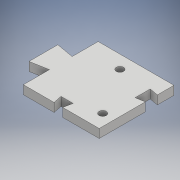
# Autodesk Inventor part: Frame VG01-04
Saved by Autodesk Inventor 2017 (Build 210142000, 142)
## iProperties
Created: 2019-03-04
Part Number: Frame VG01-04
Material: Generic
Document SubType Name: Modeling
Designer: Ben
Density: 1 g/cm^3
Appearance: Default
Author: Ben
Autodesk Inventor part; units mm, degrees
ref_plane "YZ Plane" through (0, 0, 0) normal (1, 0, 0) x (0, 1, 0)
ref_plane "XZ Plane" through (0, 0, 0) normal (0, 1, 0) x (-1, 0, 0)
ref_plane "XY Plane" through (0, 0, 0) normal (0, 0, 1) x (1, 0, 0)
sketch "Sketch1" plane through (0, 0, 0) normal (0, 1, 0) x (-1, 0, 0)
  line L0 (0, 0) -> (0, -35)
  line L1 (0, -35) -> (37, -35)
  line L2 (37, -35) -> (37, -55)
  line L3 (37, -55) -> (48, -55)
  line L4 (48, -55) -> (48, 0)
  line L5 (48, 0) -> (22, 0)
  line L6 (22, 0) -> (22, 0)
  line L7 (22, 0) -> (0, 0)
  dimension "d0" = 35
  dimension "d1" = 37
  dimension "d2" = 20
  dimension "d3" = 11
  dimension "d4" = 55
  dimension "d5" = 26
  dimension "d6" = 0
  constraints: 16 end point, 5 perpendicular, 2 vertical
  measures "d0" distance of L0.start L0.end
  measures "d1" distance of L0.end L1.end
  measures "d2" distance of L1.end L2.end
  measures "d3" distance of L2.end L3.end
  measures "d4" distance of L3.end L4.end
  measures "d5" distance of L4.end L5.end
  measures "d6" distance of L5.end L6.end
extrude "Extrusion1" add sketch "Sketch1" along normal blind 50
shell "Shell1" thickness 5 removed faces 3 at (-48, 16.6667, -36.6667) at (-19.6667, 0, -23.3333) at (-19.6667, 50, -23.3333)
sketch "Sketch2" plane through (0, 0, 0) normal (1, 0, 0) x (0, 0, -1)
  line L0 (5, 0) -> (30, 0) projected
  line L1 (5, 0) -> (19, 0)
  line L2 (19, 0) -> (19, 17)
  line L3 (19, 17) -> (5, 17)
  line L4 (5, 17) -> (5, 0)
  point P0 (0, 0)
  dimension "d10" = 17
  dimension "d11" = 0
  dimension "d12" = 11
  constraints: 8 end point, 2 parallel, 1 horizontal, 1 perpendicular, 1 point on line
  measures "d10" distance of L2.end L1.end
  measures "d11" distance from line of L4 L0.start
  measures "d12" distance from line of L2 L0.end
extrude "Extrusion2" cut sketch "Sketch2" against normal blind 10
sketch "Sketch3" plane through (-48, 0, -55) normal (-1, 0, 0) x (0, 0, 1)
  line L0 (0, 0) -> (0, 50) projected
  line L1 (5, 50) -> (25, 50) projected
  line L2 (0, 0) -> (5, 0)
  line L3 (5, 0) -> (5, 50)
  line L4 (5, 50) -> (0, 50)
  line L5 (0, 50) -> (0, 0)
  point P0 (55, 0)
  constraints: 8 end point, 2 parallel, 1 horizontal, 1 perpendicular
extrude "Extrusion3" add sketch "Sketch3" along normal blind 15
sketch "Sketch4" plane through (-48, 0, 0) normal (-1, 0, 0) x (0, 0, 1)
  line L0 (-5, 0) -> (0, 0) projected
  line L1 (-5, 0) -> (-5, 50) projected
  line L2 (0, 0) -> (-5, 0)
  line L3 (-5, 0) -> (-5, 50)
  line L4 (-5, 50) -> (0, 50)
  line L5 (0, 50) -> (0, 0)
  point P0 (0, 0)
  constraints: 8 end point, 2 parallel, 1 horizontal, 1 perpendicular
extrude "Extrusion4" add sketch "Sketch4" along normal blind 15
sketch "Sketch5" plane through (0, 17, -5) normal (0, 0, -1) x (-1, 0, 0)
  circle A0 centre (11.5, -8.5) radius 2.0828
  line L0 (63, -17) -> (0, -17) projected
  line L1 (0, -17) -> (0, 0) projected
  dimension "d19" = 4.1656
  dimension "d20" = 8.5
  dimension "d21" = 11.5
  constraints: 1 centre point
  measures "d19" diameter of A0
  measures "d20" distance from line of L0 A0.centre
  measures "d21" distance from line of L1 A0.centre
extrude "Extrusion5" cut sketch "Sketch5" against normal blind 15
sketch "Sketch6" plane through (0, 17, -5) normal (0, 0, -1) x (-1, 0, 0)
  circle A0 centre (28.505, 18.46) radius 2.0828
  line L0 (63, -17) -> (0, -17) projected
  line L1 (5, 0) -> (5, 33) projected
  dimension "d24" = 4.1656
  dimension "d25" = 35.46
  dimension "d26" = 23.505
  constraints: 1 centre point
  measures "d24" diameter of A0
  measures "d25" distance from line of L0 A0.centre
  measures "d26" distance from line of L1 A0.centre
extrude "Extrusion6" cut sketch "Sketch6" against normal blind 15
sketch "Sketch7" plane through (0, 17, -5) normal (0, 0, -1) x (-1, 0, 0)
  circle A0 centre (58.5, 19) radius 2.0828
  line L0 (63, 33) -> (63, -17) projected
  line L1 (5, 33) -> (63, 33) projected
  point P0 (0, -17)
  dimension "d29" = 4.1656
  dimension "d30" = 4.5
  dimension "d31" = 14
  constraints: 1 centre point
  measures "d29" diameter of A0
  measures "d30" distance from line of A0.centre L0
  measures "d31" distance from line of L1 A0.centre
extrude "Extrusion7" cut sketch "Sketch7" against normal blind 15
sketch "Sketch13" plane through (0, 0, -35) normal (0, 0, -1) x (-1, 0, 0)
  circle A0 centre (11.5, 8.5) radius 2.0828
  line L0 (0, 0) -> (37, 0) projected
  line L1 (0, 0) -> (0, 50) projected
  dimension "d41" = 4.1656
  dimension "d42" = 8.5
  dimension "d43" = 11.5
  constraints: 1 centre point
  measures "d41" diameter of A0
  measures "d42" distance from line of L0 A0.centre
  measures "d43" distance from line of L1 A0.centre
extrude "Extrusion9" cut sketch "Sketch13" against normal blind 15
sketch "Sketch14" plane through (-37, 0, -55) normal (0, 0, -1) x (-1, 0, 0)
  circle A0 centre (-8.495, 35.46) radius 2.0828
  line L0 (-37, 0) -> (-37, 50) projected
  line L1 (0, 0) -> (26, 0) projected
  dimension "d46" = 4.1656
  dimension "d47" = 28.505
  dimension "d48" = 35.46
  constraints: 1 centre point
  measures "d46" diameter of A0
  measures "d47" distance from line of L0 A0.centre
  measures "d48" distance from line of L1 A0.centre
extrude "Extrusion10" cut sketch "Sketch14" against normal blind 15
sketch "Sketch15" plane through (-37, 0, -55) normal (0, 0, -1) x (-1, 0, 0)
  circle A0 centre (21.5, 36) radius 2.0828
  line L0 (0, 0) -> (26, 0) projected
  line L1 (26, 50) -> (26, 0) projected
  point P0 (-37, 0)
  dimension "d51" = 4.1656
  dimension "d52" = 36
  dimension "d53" = 4.5
  constraints: 1 centre point
  measures "d51" diameter of A0
  measures "d52" distance from line of L0 A0.centre
  measures "d53" distance from line of L1 A0.centre
extrude "Extrusion11" cut sketch "Sketch15" against normal blind 15
sketch "Sketch16" plane through (-42, 0, -30) normal (-1, 0, 0) x (0, 0, 1)
  line L0 (0, 0) -> (-5, 0)
  line L1 (-5, 0) -> (-5, 50)
  line L2 (-5, 50) -> (0, 50)
  line L3 (0, 50) -> (0, 0)
  point P0 (30, 0)
  dimension "d56" = 5
  dimension "d57" = 50
  constraints: 8 end point, 2 parallel, 1 horizontal, 1 perpendicular
  measures "d56" distance of L1.end L2.end
  measures "d57" distance of L0.end L1.end
extrude "Extrusion12" add sketch "Sketch16" along normal blind 21
sketch "Sketch17" plane through (-5, 0, -30) normal (0, 0, 1) x (1, 0, 0)
  circle A0 centre (-23.505, 35.46) radius 2.0828
  line L0 (0, 0) -> (0, 50) projected
  line L1 (0, 0) -> (-58, 0) projected
  point P0 (5, 0)
  dimension "d60" = 4.1656
  dimension "d61" = 23.505
  dimension "d62" = 35.46
  constraints: 1 centre point
  measures "d60" diameter of A0
  measures "d61" distance from line of A0.centre L0
  measures "d62" distance from line of L1 A0.centre
extrude "Extrusion13" cut sketch "Sketch17" against normal blind 10
sketch "Sketch18" plane through (-42, 0, -35) normal (0, 0, -1) x (-1, 0, 0)
  circle A0 centre (16.5, 36) radius 2.0828
  line L0 (21, 50) -> (21, 0) projected
  line L1 (0, 0) -> (21, 0) projected
  point P0 (-42, 0)
  dimension "d65" = 4.1656
  dimension "d67" = 36
  dimension "d70" = 4.5
  constraints: 1 centre point
  measures "d65" diameter of A0
  measures "d67" distance from line of L1 A0.centre
  measures "d70" distance from line of L0 A0.centre
extrude "Extrusion14" cut sketch "Sketch18" against normal blind 10
sketch "Sketch20" plane through (-63, 0, 0) normal (-1, 0, 0) x (0, 0, 1)
  line L0 (0, 0) -> (-5, 0) projected
  line L1 (-5, 17) -> (-5, 50) projected
  line L2 (0, 0) -> (-5, 0)
  line L3 (-5, 0) -> (-5, 50)
  line L4 (-5, 50) -> (0, 50)
  line L5 (0, 50) -> (0, 0)
  constraints: 8 end point, 2 parallel, 1 horizontal, 1 perpendicular
extrude "Extrusion15" add sketch "Sketch20" along normal blind 2.583
sketch "Sketch21" plane through (-63, 0, -30) normal (-1, 0, 0) x (0, 0, 1)
  line L0 (-20, 50) -> (-5, 50) projected
  line L1 (11, 0) -> (0, 0) projected
  line L2 (-5, 50) -> (0, 50)
  line L3 (0, 50) -> (0, 0)
  line L4 (0, 0) -> (-5, 0)
  line L5 (-5, 0) -> (-5, 50)
  point P0 (30, 0)
  constraints: 8 end point, 2 parallel, 1 horizontal, 1 perpendicular
extrude "Extrusion16" add sketch "Sketch21" along normal blind 2.583
sketch "Sketch22" plane through (-63, 0, -55) normal (-1, 0, 0) x (0, 0, 1)
  line L0 (0, 0) -> (0, 50) projected
  line L1 (5, 0) -> (5, 50) projected
  line L2 (0, 50) -> (5, 50)
  line L3 (5, 50) -> (5, 0)
  line L4 (5, 0) -> (0, 0)
  line L5 (0, 0) -> (0, 50)
  point P0 (55, 0)
  constraints: 8 end point, 2 parallel, 1 horizontal, 1 perpendicular
extrude "Extrusion17" add sketch "Sketch22" along normal blind 2.583
sketch "Sketch23" plane through (0, 0, 0) normal (0, 0, 1) x (1, 0, 0)
  line L0 (0, 50) -> (-37, 50) projected
  line L1 (-65.583, 50) -> (-65.583, 0) projected
  line L2 (0, 50) -> (-65.583, 50)
  line L3 (-65.583, 50) -> (-65.583, 43.083)
  line L4 (-65.583, 43.083) -> (0, 43.083)
  line L5 (0, 43.083) -> (0, 50)
  point P0 (0, 0)
  dimension "d77" = 6.917
  constraints: 8 end point, 2 parallel, 1 horizontal, 1 perpendicular, 1 point on line
  measures "d77" distance of L4.end L0.start
extrude "Extrusion18" cut sketch "Sketch23" against normal blind 100
sketch "Sketch24" plane through (0, 0, -35) normal (0, 0, -1) x (-1, 0, 0)
  line L0 (0, 0) -> (65.583, 0) projected
  line L1 (31.0052, 0) -> (26.0052, 0)
  line L2 (26.0052, 5) -> (31.0052, 5)
  circle A0 centre (28.505, 35.46) radius 2.0828 projected
  line L3 (26.0052, 5) -> (25.0052, 5)
  line L4 (25.0052, 5) -> (26.0052, 0)
  line L5 (31.0052, 5) -> (32.0052, 5)
  line L6 (32.0052, 5) -> (31.0052, 0)
  dimension "d80" = 5
  dimension "d81" = 5
  dimension "d83" = 1
  dimension "d84" = 1
  constraints: 12 end point, 3 horizontal, 1 parallel, 1 point on line
  measures "d80" distance of L2.start L2.end
  measures "d81" distance of L1.end L2.start
  measures "d83" distance of L2.start L3.end
  measures "d84" distance of L2.end L5.end
extrude "Extrusion19" cut sketch "Sketch24" against normal blind 100 contours L4 L3 L2 L5 L6 L0
sketch "Sketch25" plane through (-65.583, 0, -55) normal (-1, 0, 0) x (0, 0, 1)
  line L0 (20, 0) -> (0, 0) projected
  line L1 (0, 43.083) -> (20, 43.083) projected
  line L2 (0, 0) -> (5, 0)
  line L3 (5, 0) -> (5, 43.083)
  line L4 (5, 43.083) -> (0, 43.083)
  line L5 (0, 43.083) -> (0, 0)
  point P0 (55, 0)
  dimension "d87" = 5
  constraints: 8 end point, 2 parallel, 1 horizontal, 1 perpendicular, 1 point on line
  measures "d87" distance of L4.end L3.end
extrude "Extrusion20" add sketch "Sketch25" along normal blind 22.5
sketch "Sketch28" plane through (-65.583, 0, -30) normal (-1, 0, 0) x (0, 0, 1)
  line L0 (0, 0) -> (-5, 0) projected
  line L1 (-5, 0) -> (-5, 43.083) projected
  line L2 (0, 0) -> (-5, 0)
  line L3 (-5, 0) -> (-5, 43.083)
  line L4 (-5, 43.083) -> (0, 43.083)
  line L5 (0, 43.083) -> (0, 0)
  point P0 (30, 0)
  constraints: 8 end point, 2 parallel, 1 horizontal, 1 perpendicular
extrude "Extrusion23" add sketch "Sketch28" along normal blind 22.5
sketch "Sketch26" plane through (-37, 0, -55) normal (0, 0, -1) x (-1, 0, 0)
  circle A0 centre (45.232, 36.922) radius 2.0828
  line L0 (51.083, 43.083) -> (51.083, 0) projected
  line L1 (51.083, 43.083) -> (0, 43.083) projected
  point P0 (-37, 0)
  dimension "d90" = 4.1656
  dimension "d91" = 5.851
  dimension "d92" = 6.161
  constraints: 1 centre point
  measures "d90" diameter of A0
  measures "d91" distance from line of L0 A0.centre
  measures "d92" distance from line of L1 A0.centre
extrude "Extrusion21" cut sketch "Sketch26" against normal blind 25
sketch "Sketch27" plane through (-37, 0, -55) normal (0, 0, -1) x (-1, 0, 0)
  circle A0 centre (48.381, 15.906) radius 2.0828
  line L0 (51.083, 43.083) -> (51.083, 0) projected
  line L1 (0, 0) -> (51.083, 0) projected
  point P0 (-37, 0)
  dimension "d95" = 4.1656
  dimension "d96" = 2.702
  dimension "d97" = 15.906
  constraints: 1 centre point
  measures "d95" diameter of A0
  measures "d96" distance from line of L0 A0.centre
  measures "d97" distance from line of A0.centre L1
extrude "Extrusion22" cut sketch "Sketch27" against normal blind 25
sketch "Sketch29" plane through (-42, 0, -35) normal (0, 0, -1) x (-1, 0, 0)
  circle A0 centre (43.381, 15.906) radius 2.0828 projected
  arc A1 (46.083, 19.6075) -> (46.083, 12.2045) centre (43.381, 15.906) ccw
  line L0 (46.083, 43.083) -> (46.083, 0) projected
  line L1 (46.083, 19.6075) -> (46.083, 12.2045)
  point P0 (-42, 0)
  dimension "d102" = 2.5
  constraints: 2 end point, 2 point on circle, 2 point on line, 1 centre point, 1 coincident
  measures "d102" radial gap between concentric circles of A1 A0
extrude "Extrusion24" add sketch "Sketch29" along normal up to next
sketch "Sketch30" plane through (-88.083, 0, -55) normal (-1, 0, 0) x (0, 0, 1)
  line L0 (9, 19.6075) -> (21, 19.6075)
  line L1 (21, 19.6075) -> (21, 5)
  line L2 (21, 5) -> (9, 5)
  line L3 (9, 5) -> (9, 19.6075)
  line L4 (0, 43.083) -> (0, 0) projected
  line L5 (25, 0) -> (25, 43.083) projected
  line L6 (0, 0) -> (5, 0) projected
  line L7 (20, 19.6075) -> (5, 19.6075) projected
  point P0 (55, 0)
  dimension "d105" = 9
  dimension "d106" = 4
  dimension "d107" = 5
  dimension "d108" = 0
  constraints: 8 end point, 2 parallel, 1 horizontal, 1 perpendicular
  measures "d105" distance between parallel lines of L4 L3
  measures "d106" distance between parallel lines of L5 L1
  measures "d107" distance between parallel lines of L6 L2
  measures "d108" distance between parallel lines of L7 L0
extrude "Extrusion25" add sketch "Sketch30" along normal blind 30
sketch "Sketch31" plane through (-88.083, 5, -34) normal (0, 0, 1) x (1, 0, 0)
  circle A0 centre (-23.917, 4) radius 2.0828
  line L0 (-30, 0) -> (-30, 14.6075) projected
  line L1 (0, 0) -> (-30, 0) projected
  point P0 (88.083, -5)
  dimension "d111" = 4.1656
  dimension "d112" = 6.083
  dimension "d113" = 4
  constraints: 1 centre point
  measures "d111" diameter of A0
  measures "d112" distance from line of A0.centre L0
  measures "d113" distance from line of L1 A0.centre
extrude "Extrusion26" cut sketch "Sketch31" against normal blind 30
sketch "Sketch33" plane through (-88.083, 5, -34) normal (0, 0, 1) x (1, 0, 0)
  circle A0 centre (-23.917, 4) radius 2.0828 projected
  arc A1 (-25.0228, 9.9816) -> (-30, 4) centre (-23.917, 4) ccw
  line L0 (-30, 14.6075) -> (-30, 0) projected
  line L1 (-30, 0) -> (-30, 14.6075) projected
  line L2 (0, 14.6075) -> (-30, 14.6075) projected
  line L3 (-30, 4) -> (-30, 14.6075)
  line L4 (0, 14.6075) -> (-30, 14.6075) projected
  line L5 (-30, 14.6075) -> (0, 14.6075)
  line L6 (0, 14.6075) -> (-25.0228, 9.9816)
  point P0 (88.083, -5)
  constraints: 6 end point, 2 point on circle, 2 tangent, 1 centre point, 1 coincident, 1 perpendicular, 1 point on line, 1 vertical
extrude "Extrusion27" cut sketch "Sketch33" against normal blind 30 contours A1 L0 L2 L6
sketch "Sketch34" plane through (-118.083, 5, -34) normal (0, 0, 1) x (1, 0, 0)
  circle A0 centre (6.083, 4) radius 2.0828 projected
  line L0 (0, 0) -> (0, 4) projected
  arc A1 (0, 4) -> (1.5001, 0) centre (6.083, 4) ccw
  line L1 (30, 0) -> (0, 0) projected
  line L2 (1.5001, 0) -> (0, 0)
  arc A2 (4.9772, 9.9816) -> (0, 4) centre (6.083, 4) ccw projected
  line L3 (0, 0) -> (0, 4)
  point P0 (118.083, -5)
  constraints: 4 end point, 2 point on circle, 1 centre point, 1 coincident, 1 collinear, 1 perpendicular, 1 tangent
extrude "Extrusion28" cut sketch "Sketch34" against normal blind 30 contours L0 A1 L1
sketch "Sketch35" plane through (-88.083, 5, -46) normal (0, -1, 0) x (1, 0, 0)
  line L0 (0, 12) -> (0, 11) projected
  line L1 (0, 0) -> (-28.4999, 0) projected
  line L2 (0, 11) -> (0, 0)
  line L3 (0, 0) -> (7.2848, 11)
  line L4 (7.2848, 11) -> (7.2848, -4) projected
  line L5 (0, 11) -> (7.2848, 11)
  line L6 (46.083, 11) -> (0, 11) projected
  point P0 (88.083, 46)
  constraints: 6 end point, 1 collinear, 1 perpendicular, 1 point on line
extrude "Extrusion29" add sketch "Sketch35" against normal up to next
sketch "Sketch36" plane through (0, 0, 0) normal (1, 0, 0) x (0, 0, -1)
  line L0 (30, 43.083) -> (35, 43.083) projected
  line L1 (0, 0) -> (5, 0) projected
  line L2 (30, 43.083) -> (0, 43.083)
  line L3 (0, 43.083) -> (0, 0)
  line L4 (0, 0) -> (30, 0)
  line L5 (30, 0) -> (30, 43.083)
  constraints: 8 end point, 2 parallel, 1 horizontal, 1 perpendicular
extrude "Extrusion30" cut sketch "Sketch36" against normal through all
sketch "Sketch37" plane through (0, 43.083, -35) normal (0, 0, -1) x (-1, 0, 0)
  line L0 (10, -8.694) -> (10, -17.3883)
  line L1 (10, -17.3883) -> (5, -16.5067)
  line L2 (10, -8.694) -> (5, -9.5756)
  line L3 (10, -8.694) -> (15.0771, -8.694) construction
  line L4 (5, -9.5756) -> (5, -16.5067)
  line L5 (0, -43.083) -> (0, 0) projected
  line L6 (0, -43.083) -> (26.0052, -43.083) projected
  dimension "d124" = 8.6943
  dimension "d125" = 80
  dimension "d126" = 170
  dimension "d127" = 5
  dimension "d130" = 5
  dimension "d131" = 34.389
  constraints: 10 end point, 1 equal length, 1 horizontal, 1 parallel
  measures "d124" distance of L0.start L0.end
  measures "d125" angle of L0 L1
  measures "d126" angle of L2 L3
  measures "d127" distance between parallel lines of L0 L4
  measures "d130" distance between parallel lines of L5 L4
  measures "d131" distance from line of L6 L0.start
extrude "Extrusion31" cut sketch "Sketch37" against normal blind 10
sketch "Sketch38" plane through (-37, 0, -35) normal (1, 0, 0) x (0, 0, -1)
  line L0 (20, 43.083) -> (20, 0) projected
  line L1 (0, 0) -> (20, 0)
  line L2 (20, 0) -> (20, 43.083)
  line L3 (20, 43.083) -> (0, 43.083)
  line L4 (0, 43.083) -> (0, 0)
  point P0 (-35, 0)
  constraints: 8 end point, 2 parallel, 1 horizontal, 1 perpendicular
extrude "Extrusion32" cut sketch "Sketch38" against normal through all
sketch "Sketch39" plane through (0, 0, -30) normal (1, 0, 0) x (0, 0, -1)
  line L0 (10, 34.389) -> (10, 25.6947)
  line L1 (10, 25.6947) -> (5, 26.5763)
  line L2 (10, 34.389) -> (5, 33.5074)
  line L3 (10, 34.389) -> (15.0771, 34.389) construction
  line L4 (5, 33.5074) -> (5, 26.5763)
  line L5 (5, 0) -> (5, 43.083) projected
  point P0 (5, 33.5074)
  dimension "d136" = 8.6943
  dimension "d137" = 80
  dimension "d138" = 170
  dimension "d139" = 5
  dimension "d140" = 0
  dimension "d141" = 8.694
  constraints: 10 end point, 1 equal length, 1 horizontal, 1 parallel
  measures "d136" distance of L0.start L0.end
  measures "d137" angle of L0 L1
  measures "d138" angle of L2 L3
  measures "d139" distance between parallel lines of L0 L4
  measures "d140" distance between parallel lines of L5 L4
  measures "d141" vertical distance of L5.end L0.start
extrude "Extrusion33" add sketch "Sketch39" against normal blind 42
sketch "Sketch40" plane through (0, 0, -30) normal (1, 0, 0) x (0, 0, -1)
  line L0 (5, 38.0828) -> (5, 33.9172) projected
  line L1 (5, 36.5278) -> (10.9453, 36.5278)
  line L2 (10.9453, 36.5278) -> (10.9453, 22.5092)
  line L3 (10.9453, 22.5092) -> (5, 22.5092)
  line L4 (5, 22.5092) -> (5, 36.5278)
  point P0 (-30, 0)
  constraints: 8 end point, 2 parallel, 1 horizontal, 1 perpendicular, 1 point on line
extrude "Extrusion34" cut sketch "Sketch40" against normal blind 37
sketch "Sketch41" plane through (0, 0, -35) normal (0, 0, -1) x (-1, 0, 0)
  line L0 (0, 0) -> (5, 0)
  line L1 (5, 0) -> (5, 45.0451)
  line L2 (5, 45.0451) -> (0, 45.0451)
  line L3 (0, 45.0451) -> (0, 0)
  dimension "d146" = 5
  constraints: 8 end point, 2 parallel, 1 horizontal, 1 perpendicular
  measures "d146" distance of L2.end L1.end
extrude "Extrusion35" cut sketch "Sketch41" against normal blind 27
sketch "Sketch43" plane through (-37, 0, -30) normal (1, 0, 0) x (0, 0, -1)
  line L0 (10, 16.9997) -> (10, 8.3054)
  line L1 (10, 8.3054) -> (5, 9.187)
  line L2 (10, 16.9997) -> (5, 16.118)
  line L3 (10, 16.9997) -> (15.0771, 16.9997) construction
  line L4 (5, 16.118) -> (5, 9.187)
  line L5 (10, 34.389) -> (10, 25.6947) projected
  point P0 (5, 0)
  dimension "d149" = 8.6943
  dimension "d150" = 80
  dimension "d151" = 170
  dimension "d152" = 5
  dimension "d153" = 0
  dimension "d154" = 9.187
  constraints: 10 end point, 1 equal length, 1 horizontal, 1 parallel
  measures "d149" distance of L0.start L0.end
  measures "d150" angle of L0 L1
  measures "d151" angle of L2 L3
  measures "d152" distance between parallel lines of L0 L4
  measures "d153" distance between parallel lines of L5 L0
  measures "d154" distance of point (5, 0) L1.end
extrude "Extrusion36" add sketch "Sketch43" against normal blind 5
sketch "Sketch44" plane through (-25.0052, 5, -35) normal (0, 0, -1) x (-1, 0, 0)
  line L0 (23.6844, 38.083) -> (23.6844, 23.083)
  line L1 (23.6844, 23.083) -> (33.6844, 24.8463)
  line L2 (33.6844, 24.8463) -> (33.6844, 8.2367)
  line L3 (33.6844, 8.2367) -> (23.6844, 10)
  line L4 (23.6844, 10) -> (23.6844, -5)
  line L5 (6, -5) -> (63.0778, -5) projected
  line L6 (63.0778, 38.083) -> (-20.0052, 38.083) projected
  line L7 (23.6844, 38.083) -> (96.1703, 54.1884)
  line L8 (96.1703, 54.1884) -> (94.0332, -32.3639)
  line L9 (94.0332, -32.3639) -> (23.6844, -5)
  point P0 (-25.0052, -5)
  dimension "d157" = 15
  dimension "d158" = 15
  dimension "d159" = 13.083
  dimension "d160" = 80
  dimension "d161" = 80
  dimension "d162" = 10
  constraints: 16 end point, 3 point on line, 1 parallel, 1 perpendicular, 1 vertical
  measures "d157" distance of L3.end L4.end
  measures "d158" distance of L0.start L0.end
  measures "d159" distance of L3.end L0.end
  measures "d160" angle of L4 L3
  measures "d161" angle of L0 L1
  measures "d162" distance between parallel lines of L0 L2
extrude "Extrusion37" cut sketch "Sketch44" against normal through all
body "Solid1"
